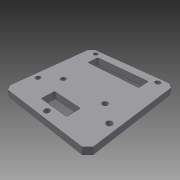
# Autodesk Inventor part: x_carriage
Saved by Autodesk Inventor 2014 (Build 180170000, 170)
## iProperties
Created: 2013-11-06
Part Number: x_carriage
Material: Generic
Document SubType Name: Modeling
Designer: buben
Density: 1 g/cm^3
Appearance: Default
Author: buben
Subject: Laser Cutted
Autodesk Inventor part; units mm, degrees
ref_plane "YZ Plane" through (0, 0, 0) normal (1, 0, 0) x (0, 1, 0)
ref_plane "XZ Plane" through (0, 0, 0) normal (0, 1, 0) x (-1, 0, 0)
ref_plane "XY Plane" through (0, 0, 0) normal (0, 0, 1) x (1, 0, 0)
sketch "Sketch1" plane through (0, 0, 0) normal (0, 0, 1) x (1, 0, 0)
  line L0 (4, 0) -> (76, 0)
  line L1 (80, 4) -> (80, 79.5)
  line L2 (76, 83.5) -> (4, 83.5)
  line L3 (0, 79.5) -> (0, 4)
  line L4 (0, 4) -> (4, 0)
  line L5 (76, 0) -> (80, 4)
  line L6 (80, 79.5) -> (76, 83.5)
  line L7 (4, 83.5) -> (0, 79.5)
  line L8 (16.5, 75) -> (63.5, 75)
  line L9 (64.5, 74) -> (64.5, 65)
  line L10 (63.5, 64) -> (16.5, 64)
  line L11 (15.5, 65) -> (15.5, 74)
  arc A0 (15.5, 65) -> (16.5, 64) centre (16.5, 65) ccw
  arc A1 (16.5, 75) -> (15.5, 74) centre (16.5, 74) ccw
  arc A2 (64.5, 74) -> (63.5, 75) centre (63.5, 74) ccw
  arc A3 (63.5, 64) -> (64.5, 65) centre (63.5, 65) ccw
  line L12 (28.5, 21) -> (51.5, 21)
  line L13 (52.5, 20) -> (52.5, 11)
  line L14 (51.5, 10) -> (28.5, 10)
  line L15 (27.5, 11) -> (27.5, 20)
  arc A4 (27.5, 11) -> (28.5, 10) centre (28.5, 11) ccw
  arc A5 (28.5, 21) -> (27.5, 20) centre (28.5, 20) ccw
  arc A6 (52.5, 20) -> (51.5, 21) centre (51.5, 20) ccw
  arc A7 (51.5, 10) -> (52.5, 11) centre (51.5, 11) ccw
  line L16 (15.5, 69.5) -> (64.5, 69.5) construction
  line L17 (27.5, 15.5) -> (52.5, 15.5) construction
  circle A8 centre (40, 5) radius 2.25
  circle A9 centre (10, 78.5) radius 2.25
  circle A10 centre (6, 23.25) radius 2.25
  circle A11 centre (74, 23.25) radius 2.25
  circle A12 centre (70, 78.5) radius 2.25
  point P0 (0, 0)
  point P1 (40, 64)
  point P2 (40, 21)
  point P3 (40, 75)
  point P4 (40, 83.5)
  point P5 (0, 41.75)
  point P6 (80, 41.75)
  dimension "d0" = 45
  dimension "d1" = 4
  dimension "d2" = 1
  dimension "d3" = 11
  dimension "d4" = 49
  dimension "d5" = 1
  dimension "d6" = 11
  dimension "d7" = 25
  dimension "d9" = 10
  dimension "d10" = 8.5
  dimension "d11" = 4.5
  dimension "d12" = 4.5
  dimension "d13" = 5
  dimension "d14" = 5
  dimension "d15" = 4.5
  dimension "d16" = 4.5
  dimension "d19" = 54
  dimension "d22" = 80
  dimension "d23" = 6
  dimension "d24" = 6
  dimension "d25" = 23.25
  dimension "d26" = 4.5
  dimension "d27" = 10
  dimension "d28" = 10
  constraints: 36 end point, 16 point on circle, 16 tangent, 13 centre point, 10 midpoint, 10 vertical alignment, 8 horizontal alignment, 8 parallel, 4 perpendicular, 3 horizontal
  measures "d0" angle of L0 L4
  measures "d1" horizontal distance of L0.start L3.end
  measures "d2" radius of A1
  measures "d3" distance of L10.start L8.end
  measures "d4" distance of L11.end L9.start
  measures "d5" radius of A5
  measures "d6" distance of L14.start L12.end
  measures "d7" distance of L15.end L13.start
  measures "d9" distance from line of L0 L14.end
  measures "d10" distance from line of L2 L8.start
  measures "d11" diameter of A8
  measures "d12" diameter of A9
  measures "d13" distance from line of L0 A8.centre
  measures "d14" distance from line of L2 A9.centre
  measures "d15" diameter of A10
  measures "d16" diameter of A11
  measures "d19" distance between parallel lines of L17 L16
  measures "d22" distance between parallel lines of L3 L1
  measures "d23" distance from line of L3 A10.centre
  measures "d24" distance from line of L1 A11.centre
  measures "d25" distance from line of L0 A10.centre
  measures "d26" diameter of A12
  measures "d27" distance from line of L3 A9.centre
  measures "d28" distance from line of L1 A12.centre
extrude "Extrusion2" add sketch "Sketch1" along normal blind 6
sketch "Sketch2" plane through (0, 0, 6) normal (0, 0, 1) x (1, 0, 0)
  line L0 (4, 0) -> (76, 0) projected
  circle A0 centre (20, 35) radius 2.25
  circle A1 centre (60, 35) radius 2.25
  line L1 (20, 35) -> (60, 35) construction
  point P0 (0, 0)
  point P1 (40, 35)
  point P2 (40, 0)
  dimension "d31" = 4.5
  dimension "d32" = 4.5
  dimension "d33" = 40
  dimension "d34" = 35
  constraints: 2 centre point, 2 end point, 2 midpoint, 1 horizontal alignment, 1 parallel, 1 vertical alignment
  measures "d31" diameter of A1
  measures "d32" diameter of A0
  measures "d33" distance of L1.end L1.start
  measures "d34" distance from line of L0 L1.end
extrude "Extrusion3" cut sketch "Sketch2" against normal through all
body "Solid2"
